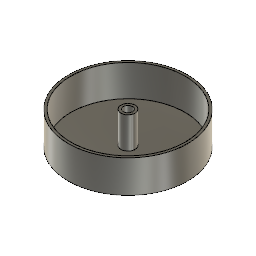
motor_moat (Autodesk Fusion 360 design; units mm, degrees)
Autodesk Fusion 360 part; units mm, degrees
sketch "Sketch1" plane through (0, 0, 0) normal (0, 0, 1) x (1, 0, 0)
  circle A0 centre (0, 0) radius 47.5
  dimension "d1" = 95
  constraint coincident A0.centre origin
  measures "d1" diameter of A0
extrude "Extrude1" add sketch "Sketch1" along normal blind 1
sketch "Sketch2" plane through (0, 0, 1) normal (0, 0, 1) x (-1, 0, 0)
  circle A0 centre (0, 0) radius 47.5
  circle A1 centre (0, 0) radius 45.5
  circle A2 centre (0, 0) radius 32.5
  dimension "d4" = 91
  dimension "d5" = 65
  constraint coincident A0.centre A1.centre
  measures "d4" diameter of A1
  measures "d5" diameter of A2
extrude "Extrude2" add sketch "Sketch2" along normal blind 25 contours A0
sketch "Sketch5" plane through (0, 0, 1) normal (0, 0, 1) x (-1, 0, 0)
  circle A0 centre (0, 0) radius 45.5
  circle A1 centre (0, 0) radius 3.65
  circle A2 centre (0, 0) radius 5.6
  dimension "d16" = 7.3
  dimension "d17" = 11.2
  constraint coincident A0.centre A1.centre
  constraint concentric A1 A2
  measures "d16" diameter of A1
  measures "d17" diameter of A2
extrude "Extrude5" add sketch "Sketch5" along normal blind 25 contours A2
extrude "Extrude6" cut 1 faces at (0.8126, 0.5926, 1) along direction (0, 0, -1) blind 1
